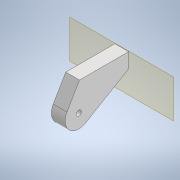
# Autodesk Inventor part: pivot module stalk
Saved by Autodesk Inventor 2022 (Build 260153000, 153)
## iProperties
Created: 2021-12-08
Part Number: pivot module stalk
Material: Generic
Document SubType Name: Modeling
Designer: efred
Density: 1 g/cm^3
Appearance: Default
Author: efred
Autodesk Inventor part; units mm, degrees
ref_plane "YZ Plane" through (0, 0, 0) normal (1, 0, 0) x (0, 1, 0)
ref_plane "XZ Plane" through (0, 0, 0) normal (0, 1, 0) x (-1, 0, 0)
ref_plane "XY Plane" through (0, 0, 0) normal (0, 0, 1) x (1, 0, 0)
ref_plane "Work Plane1" through (0, 0, 0) normal (0, 0, 1) x (1, 0, 0)
sketch "Sketch1" plane through (0, 0, 0) normal (0, 0, 1) x (1, 0, 0)
  circle A0 centre (0, 7.1) radius 1.5 projected
  circle A1 centre (3, 11.1) radius 1.5
  circle A2 centre (-3, 11.1) radius 1.5
  line L0 (-5.8, -25.5252) -> (-5.8, 18.8938) projected
  line L1 (-5.8, 18.8938) -> (5.8, 18.8938) projected
  line L2 (5.8, 18.8938) -> (5.8, -25.5252) projected
  line L3 (-5.6, 3.1) -> (5.6, 3.1)
  line L4 (5.6, 3.1) -> (5.6, 15.1)
  line L5 (5.6, 15.1) -> (-5.6, 15.1)
  line L6 (-5.6, 15.1) -> (-5.6, 3.1)
  line L7 (0, 7.1) -> (0, 6.0369) construction
  point P0 (0, 0)
  dimension "d0" = 0.2
  dimension "d1" = 0.2
  dimension "d3" = 4
  dimension "d4" = 4
  dimension "d10" = 4
  dimension "d11" = 3
  dimension "d12" = 3
  constraints: 10 end point, 2 centre point, 2 parallel, 1 horizontal, 1 perpendicular, 1 vertical, 1 other
  measures "d0" distance between parallel lines of L2 L4
  measures "d1" distance between parallel lines of L0 L6
  measures "d3" distance from line of L7.start L3
  measures "d4" distance from line of A1.centre L5
  measures "d10" vertical distance of L7.start A1.centre
  measures "d11" horizontal distance of L7.start A1.centre
  measures "d12" diameter of A1
extrude "Extrusion1" add sketch "Sketch1" along normal blind 40
sketch "Sketch2" plane through (5.6, 3.1, 0) normal (1, 0, 0) x (0, 0, -1)
  circle A0 centre (-40.6, -11.1) radius 2.05 construction
  line L0 (-40, 0) -> (-40, 12) projected
  circle A1 centre (-40.6, -11.1) radius 11.1162
  line L1 (-40, 12) -> (-50.2033, -5.5012)
  line L2 (0, 0) -> (-40, 0) projected
  circle A2 centre (-40.6, -11.1) radius 2.15
  line L3 (-33.0963, -19.3015) -> (-12, 0)
  point P0 (0, -3.1)
  dimension "d7" = 4.3
  dimension "d14" = 12
  constraints: 4 end point, 3 point on circle, 2 centre point, 2 tangent, 1 coincident, 1 concentric, 1 point on line
  measures "d7" diameter of A2
  measures "d14" distance of L3.end L2.start
extrude "Extrusion2" add sketch "Sketch2" against normal up to surface (11.2 mm away)
body "Solid1"
